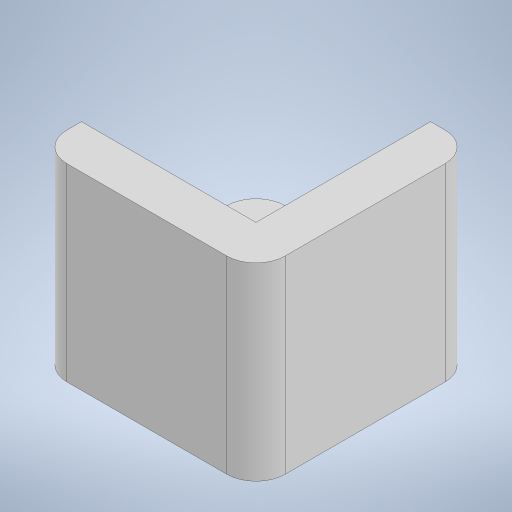
# Autodesk Inventor part: legs
Saved by Autodesk Inventor 2024 (Build 280153000, 153)
## iProperties
Created: 2026-03-15
Part Number: legs
Material: Generic
Document SubType Name: Modeling
Designer: HP
Density: 1 g/cm^3
Appearance: Default
Author: HP
Autodesk Inventor part; units mm, degrees
ref_plane "YZ Plane" through (0, 0, 0) normal (1, 0, 0) x (0, 1, 0)
ref_plane "XZ Plane" through (0, 0, 0) normal (0, 1, 0) x (-1, 0, 0)
ref_plane "XY Plane" through (0, 0, 0) normal (0, 0, 1) x (1, 0, 0)
sketch "Sketch1" plane through (0, 0, 0) normal (0, 1, 0) x (-1, 0, 0)
  line L0 (0, 0) -> (0, 7.5)
  line L1 (0, 7.5) -> (7.5, 7.5)
  line L2 (7.5, 7.5) -> (7.5, -7.5)
  line L3 (7.5, -7.5) -> (-7.5, -7.5)
  line L4 (-7.5, -7.5) -> (-7.5, 7.5)
  line L5 (-7.5, 7.5) -> (0, 7.5)
  dimension "d0" = 7.5
  dimension "d1" = 7.5
  dimension "d2" = 15
  dimension "d3" = 15
  constraints: 12 end point, 5 perpendicular, 1 point on line, 1 vertical
  measures "d0" distance of L0.start L0.end
  measures "d1" distance of L0.end L1.end
  measures "d2" distance of L1.end L2.end
  measures "d3" distance of L2.end L3.end
extrude "Extrusion1" add sketch "Sketch1" along normal blind 3
fillet "Fillet1" radius 2 4 edges at (7.5, 1.5, 7.5) (7.5, 1.5, -7.5) (-7.5, 1.5, 7.5) (-7.5, 1.5, -7.5)
sketch "Sketch2" plane through (0, 3, 0) normal (0, 1, 0) x (1, 0, 0)
  circle A0 centre (0, 0) radius 2
  dimension "d7" = 4
  constraints: 1 centre point, 1 coincident
  measures "d7" diameter of A0
extrude "Extrusion2" cut sketch "Sketch2" against normal blind 3
sketch "Sketch3" plane through (0, 3, 0) normal (0, 1, 0) x (1, 0, 0)
  line L0 (0, 0) -> (7.5, 0)
  line L1 (7.5, -5.5) -> (7.5, 5.5) projected
  line L2 (7.5, 0) -> (4.5, 0)
  line L3 (4.5, 0) -> (4.5, 4.5)
  line L4 (4.5, 4.5) -> (4.5, -4.5)
  line L5 (4.5, -4.5) -> (-4.5, -4.5)
  line L6 (-4.5, -4.5) -> (-7.5, -4.5)
  line L7 (-7.5, 5.5) -> (-7.5, -5.5) projected
  line L8 (4.5, 4.5) -> (4.5, 7.5)
  line L9 (5.5, 7.5) -> (-5.5, 7.5) projected
  line L10 (4.5, 7.5) -> (5.5, 7.5)
  line L11 (7.5, 5.5) -> (7.5, -5.5)
  line L12 (-5.5, -7.5) -> (5.5, -7.5) projected
  line L13 (5.5, -7.5) -> (-5.5, -7.5)
  arc A0 (7.5, 5.5) -> (5.5, 7.5) centre (5.5, 5.5) ccw projected
  arc A1 (7.5, 5.5) -> (5.5, 7.5) centre (5.5, 5.5) ccw
  arc A2 (5.5, -7.5) -> (7.5, -5.5) centre (5.5, -5.5) ccw projected
  arc A3 (5.5, -7.5) -> (7.5, -5.5) centre (5.5, -5.5) ccw
  line L14 (-7.5, -4.5) -> (-7.5, -5.5)
  arc A4 (-7.5, -5.5) -> (-5.5, -7.5) centre (-5.5, -5.5) ccw projected
  arc A5 (-7.5, -5.5) -> (-5.5, -7.5) centre (-5.5, -5.5) ccw
  dimension "d10" = 3
  dimension "d11" = 4.5
  dimension "d12" = 9
  dimension "d13" = 9
  dimension "d14" = 3
  constraints: 22 end point, 6 point on circle, 5 point on line, 3 centre point, 2 collinear, 2 vertical, 1 concentric, 1 midpoint, 1 perpendicular, 1 tangent
  measures "d10" distance of L0.end L2.end
  measures "d11" distance of L2.end L3.end
  measures "d12" distance of L3.end L4.end
  measures "d13" distance of L4.end L5.end
  measures "d14" distance of L3.end L8.end
extrude "Extrusion3" add sketch "Sketch3" along normal blind 10
body "Solid1"
